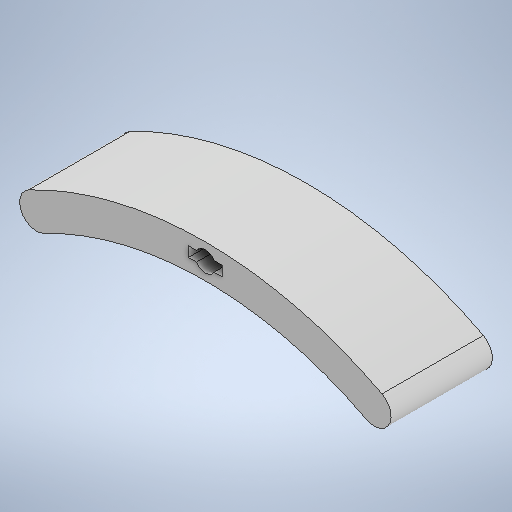
# Autodesk Inventor part: Part5
Saved by Autodesk Inventor 2025.4 (Build 294407000, 407)
## iProperties
Created: 2026-03-03
Part Number: Part5
Material: Generic
Document SubType Name: Modeling
Designer: Amir
Density: 1 g/cm^3
Appearance: Default
Author: Amir
Autodesk Inventor part; units mm, degrees
ref_plane "YZ Plane" through (0, 0, 0) normal (1, 0, 0) x (0, 1, 0)
ref_plane "XZ Plane" through (0, 0, 0) normal (0, 1, 0) x (-1, 0, 0)
ref_plane "XY Plane" through (0, 0, 0) normal (0, 0, 1) x (1, 0, 0)
sketch "Sketch1" plane through (0, 0, 0) normal (0, 0, 1) x (1, 0, 0)
  arc A0 (25, 5.7414) -> (-25, 5.7414) centre (0, -42.123) ccw construction
  arc A1 (26.1574, 7.9574) -> (-26.1574, 7.9574) centre (0, -42.123) ccw
  arc A2 (23.8426, 3.5255) -> (-23.8426, 3.5255) centre (0, -42.123) ccw
  arc A3 (23.8426, 3.5255) -> (26.1574, 7.9574) centre (25, 5.7414) ccw
  arc A4 (-26.1574, 7.9574) -> (-23.8426, 3.5255) centre (-25, 5.7414) ccw
  line L0 (2.5, 11.127) -> (2.5, 12.627)
  line L1 (-2.5, 12.627) -> (-2.5, 11.127)
  arc A5 (-1.299, 11.127) -> (1.299, 11.127) centre (0, 11.877) ccw
  arc A6 (1.299, 12.627) -> (-1.299, 12.627) centre (0, 11.877) ccw
  line L2 (2.5, 12.627) -> (1.299, 12.627)
  line L3 (-1.299, 12.627) -> (-2.5, 12.627)
  line L4 (-2.5, 11.127) -> (-1.299, 11.127)
  line L5 (1.299, 11.127) -> (2.5, 11.127)
  point P0 (0, 0)
  dimension "d1" = 50
  dimension "d2" = 54
  dimension "d3" = 5
  dimension "d5" = 5
  dimension "d7" = 1.5
  dimension "d9" = 1.5
  dimension "d10" = 51.5
  dimension "d11" = 56.5
  constraints: 15 point on circle, 12 end point, 7 centre point, 5 parallel, 4 tangent, 2 horizontal, 2 perpendicular, 1 vertical alignment
  measures "d1" distance of A4.centre A0.start
  measures "d2" radius of A0
  measures "d3" diameter of A3
  measures "d5" distance of L1.start L0.end
  measures "d7" distance of L0.start L0.end
  measures "d9" radius of A6
  measures "d10" radius of A2
  measures "d11" radius of A1
extrude "Extrusion1" add sketch "Sketch1" along normal blind 15
body "Solid1"
